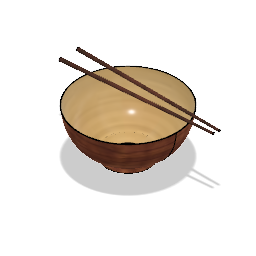
17-Day 11 - Japanese Bowl and Chopsticks v2 (Autodesk Fusion 360 design; units mm, degrees)
Autodesk Fusion 360 part; units mm, degrees
sketch "Sketch1" plane through (0, 0, 0) normal (0, 0, 1) x (1, 0, 0)
  line L0 (0, 0) -> (20, 0)
  line L1 (20, 0) -> (20, 10)
  line L2 (0, 1) -> (19, 1)
  line L3 (19, 1) -> (19, 10)
  line L4 (0, 0) -> (0, 1)
  line L5 (82, 80) -> (80.9948, 80)
  spline S0 degree 3 poles (19.7622, 10.9713) (31.2698, 13.7891) (41.4067, 17.7408) (49.8853, 23.0341) (57.0121, 27.4835) (62.9167, 32.9157) (67.5252, 39.4564) (74, 48.6458) (78.0037, 59.9892) (80.084, 73.0167) (80.4474, 75.2927) (80.7509, 77.6206) (80.9948, 80) knots 0 0 0 0 0.309524 0.309524 0.309524 0.5697 0.5697 0.5697 0.935235 0.935235 0.935235 0.999095 0.999095 0.999095 0.999095
  line L6 (19, 10) -> (0, 10)
  line L7 (0, 10) -> (0, 11)
  line L8 (0, 11) -> (19.7622, 10.9713)
  line L9 (20, 0) -> (36, 0)
  line L10 (20, 1) -> (35, 1)
  line L11 (49, 21.3241) -> (49, 21.9287)
  line L12 (40, 0) -> (40, 1)
  line L13 (35, 1) -> (35, 14.6351)
  line L14 (36, 0) -> (36, 15.0232)
  spline S1 degree 5 poles (20, 10) (22.2463, 10.55) (25.3609, 11.3802) (28.388, 12.2843) (31.3264, 13.2634) (34.1739, 14.3192) (35, 14.6351) knots 0 0 0 0 0 0 0.1 0.141416 0.141416 0.141416 0.141416 0.141416 0.141416
  line L15 (33.5502, 14.0807) -> (36.4498, 15.1894)
  spline S2 degree 5 poles (36, 15.0232) (36.9586, 15.4007) (39.8599, 16.5847) (44.5427, 18.7113) (50.6915, 22.047) (57.794, 27.0245) (64.5887, 33.5222) (70.2105, 41.0106) (74.7026, 49.4532) (78.1489, 58.7791) (80.1373, 66.8891) (81.2236, 73.3137) (81.7707, 77.7463) (82, 80) knots 0.15149 0.15149 0.15149 0.15149 0.15149 0.15149 0.2 0.3 0.4 0.5 0.6 0.7 0.8 0.9 1 1 1 1 1 1
  line L16 (26.5921, 11.3175) -> (45.4079, 18.7288)
  point P0 (64.5, 34)
  dimension "d4" = -1
  constraint coincident L0.start L4.start
  constraint horizontal L0
  constraint perpendicular L0 L1
  constraint perpendicular L2 L4
  constraint perpendicular L3 L6
  constraint perpendicular L6 L7
  constraint perpendicular L1 L9
  constraint parallel L9 L10
  constraint coincident L11.start S2
  constraint perpendicular L10 L12
  constraint perpendicular L10 L13
  constraint perpendicular L10 L14
  constraint midpoint L13.end L15
  constraint midpoint L14.end L16
revolve "Revolve1" add sketch "Sketch1" angle 360 about axis through (0, 1.75, 0) along (0, 1, 0) contours L0 L1 L2 L3 L4 L5 S0 L6 L7 L8 S1 L15 S2 L16 | L1 L9 L10 L13 L14 L15 L16 | L14 L15 L16 | L13 L15 L16 makes body 1
sketch "Sketch2" plane through (0, 0, 0) normal (1, 0, 0) x (0, 0, -1)
  circle A0 centre (35, 100) radius 2
  dimension "d5" = 4
  measures "d5" diameter of A0
ref_plane "WorkPlane1" through (-240, 0, 0) normal (1, 0, 0) x (0, 1, 0)
sketch "Sketch3" plane through (-240, 0, 0) normal (1, 0, 0) x (0, 0, -1)
  circle A0 centre (35, 100) radius 3
  dimension "d7" = 6
  measures "d7" diameter of A0
loft "Loft1" add profiles "Sketch3", "Sketch2" section 1 section 2 separate body makes body 2
move_body "Move1" bodies 2 to x (1, 0, 0) y (0, 1, 0) z (0, 0, 1) at (120, -15, 0)
copy_body "CopyPasteBodies1" bodies 2 makes body 3
move_body "Move2" bodies 3 to x (0.996195, 0, -0.087156) y (0, 1, 0) z (0.087156, 0, 0.996195) at (2.5938, 0, 19.4081)
extrude "Extrude1" cut 2 faces at (-3.277, 0, 1.2855) (-30.5044, 0, 0) along direction (0, 1, 0) blind 5 on bodies 1 bodies 1
sketch "Sketch4" plane through (0, 5, 0) normal (0, -1, 0) x (1, 0, 0)
  circle A0 centre (0, 0) radius 36
  circle A1 centre (0, 0) radius 35
  circle A2 centre (0, 0) radius 36
  constraint coincident A0.centre A1.centre
extrude "Extrude2" add sketch "Sketch4" against normal blind 2 contours A1 bodies 1
